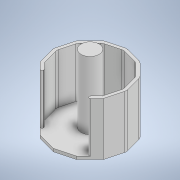
# Autodesk Inventor part: holder-12
Saved by Autodesk Inventor 2020 (Build 240168000, 168)
## iProperties
Created: 2020-02-17
Part Number: holder-12
Material: Generic
Document SubType Name: Modeling
Designer: Ball
Density: 1 g/cm^3
Appearance: Default
Author: Ball
Autodesk Inventor part; units mm, degrees
ref_plane "YZ Plane" through (0, 0, 0) normal (1, 0, 0) x (0, 1, 0)
ref_plane "XZ Plane" through (0, 0, 0) normal (0, 1, 0) x (-1, 0, 0)
ref_plane "XY Plane" through (0, 0, 0) normal (0, 0, 1) x (1, 0, 0)
sketch "Sketch1" plane through (0, 0, 0) normal (0, 1, 0) x (-1, 0, 0)
  line L0 (52.592, 0) -> (45.546, -26.296)
  line L1 (45.546, -26.296) -> (26.296, -45.546)
  line L2 (26.296, -45.546) -> (0, -52.592)
  line L3 (0, -52.592) -> (-26.296, -45.546)
  line L4 (-26.296, -45.546) -> (-45.546, -26.296)
  line L5 (-45.546, -26.296) -> (-52.592, 0)
  line L6 (-52.592, 0) -> (-45.546, 26.296)
  line L7 (-45.546, 26.296) -> (-26.296, 45.546)
  line L8 (-26.296, 45.546) -> (0, 52.592)
  line L9 (0, 52.592) -> (26.296, 45.546)
  line L10 (26.296, 45.546) -> (45.546, 26.296)
  line L11 (45.546, 26.296) -> (52.592, 0)
  point P0 (0, 0)
  point P1 (0, 0)
  dimension "d0" = 50.8
  constraints: 24 end point, 1 coincident, 25 other
  measures "d0" distance from line of L2 point (0, 0)
extrude "Extrusion1" add sketch "Sketch1" along normal blind 76.2
sketch "Sketch2" plane through (0, 76.2, 0) normal (0, 1, 0) x (1, 0, 0)
  line L0 (-48.1743, 0) -> (-41.7202, 24.0871)
  line L1 (-41.7202, 24.0871) -> (-24.0871, 41.7202)
  line L2 (-24.0871, 41.7202) -> (0, 48.1743)
  line L3 (0, 48.1743) -> (24.0871, 41.7202)
  line L4 (24.0871, 41.7202) -> (41.7202, 24.0871)
  line L5 (41.7202, 24.0871) -> (48.1743, 0)
  line L6 (48.1743, 0) -> (41.7202, -24.0871)
  line L7 (41.7202, -24.0871) -> (32.9037, -32.9037)
  line L8 (-32.9037, -32.9037) -> (-41.7202, -24.0871)
  line L9 (-41.7202, -24.0871) -> (-48.1743, 0)
  line L10 (-52.592, 0) -> (-45.546, -26.296) projected
  line L11 (-32.9037, -32.9037) -> (-32.9037, -66.8246)
  line L12 (-32.9037, -66.8246) -> (32.9037, -66.8246)
  line L13 (32.9037, -66.8246) -> (32.9037, -32.9037)
  point P0 (0, 0)
  point P1 (0, 0)
  dimension "d3" = 4.2672
  constraints: 26 end point, 2 perpendicular, 1 coincident, 1 vertical, 18 other
  measures "d3" distance between parallel lines of L10 L9
extrude "Extrusion2" cut sketch "Sketch2" against normal blind 71.9328
fillet "Fillet1" radius 1.905 4 edges at (-32.9037, 40.2336, 38.9384) (-32.9037, 40.2336, 32.9037) (32.9037, 40.2336, 38.9384) (32.9037, 40.2336, 32.9037)
sketch "Sketch3" plane through (0, 4.2672, 0) normal (0, 1, 0) x (1, 0, 0)
  circle A0 centre (0, 0) radius 12.954
  dimension "d7" = 25.908
  constraints: 1 centre point, 1 coincident
  measures "d7" diameter of A0
extrude "Extrusion3" add sketch "Sketch3" along normal blind 97.3328
fillet "Fillet2" radius 8.89 14 edges at (52.592, 38.1, 0) (45.546, 38.1, -26.296) (26.296, 38.1, -45.546) (0, 38.1, -52.592) (-26.296, 38.1, -45.546) (-45.546, 38.1, -26.296) (-52.592, 38.1, 0) (-48.1743, 40.2336, 0) (-41.7202, 40.2336, -24.0871) (-24.0871, 40.2336, -41.7202) (0, 40.2336, -48.1743) (24.0871, 40.2336, -41.7202) (41.7202, 40.2336, -24.0871) (48.1743, 40.2336, 0)
body "Solid1"
